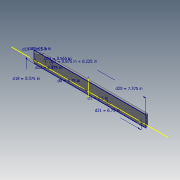
# Autodesk Inventor part: FLUGGER CAP SIDE FLUSH GUIDE
Saved by Autodesk Inventor 2020.3 (Build 243373000, 373)
## iProperties
RuleStatus: InUse
AfterDocSave0: file://Part Number Cleaner
Created: 2018-10-13
Material: Generic
Vendor: HHMI: JRC - ID&F
Document SubType Name: Modeling
Designer: arnoldj
Density: 1 g/cm^3
Appearance: Default
DESIGN DEPARTMENT: HHMI: JRC - ID&F
ALTERED ITEM PART NUMBER: N/A
ALTERED ITEM VENDOR: N/A
ALTERED ITEM DESCRIPTION: N/A
Author: arnoldj
Revision Number: 0
Autodesk Inventor part; units mm, degrees
ref_plane "YZ Plane" through (0, 0, 0) normal (1, 0, 0) x (0, 1, 0)
ref_plane "XZ Plane" through (0, 0, 0) normal (0, 1, 0) x (-1, 0, 0)
sketch "Sketch1" plane through (0, 0, 0) normal (0, 0, 1) x (1, 0, 0)
  line L0 (0, 35.433) -> (0, -17.018) projected
  line L1 (-250.825, 0) -> (260.35, 0) projected
  line L2 (187.325, -9.525) -> (-177.8, -9.525)
  line L3 (-177.8, -9.525) -> (-177.8, 27.94)
  line L4 (-177.8, 27.94) -> (187.325, 27.94)
  line L5 (187.325, 27.94) -> (187.325, -9.525)
  point P0 (0, 0)
  point P1 (-171.45, 0)
  point P2 (0, 0)
  point P3 (63.5, 0)
  point P4 (171.45, 0)
  point P5 (-139.7, 13.589)
  point P6 (-117.475, 13.589)
  dimension "d0" = 171.45
  dimension "d1" = 63.5
  dimension "d17" = 27.94
  dimension "d18" = 9.525
  dimension "d19" = 6.35
  dimension "d20" = 187.325
  dimension "d21" = 171.45
  dimension "d33" = 22.225
  dimension "d34" = 14.351
  dimension "d35" = 38.1
  constraints: 8 end point, 5 point on line, 2 parallel, 1 horizontal, 1 horizontal alignment, 1 perpendicular
  measures "d0" distance from line of L0 point (-171.45, 0)
  measures "d1" distance from line of L0 point (63.5, 0)
  measures "d17" distance between parallel lines of L1 L4
  measures "d18" distance between parallel lines of L2 L1
  measures "d19" distance from line of point (-171.45, 0) L3
  measures "d20" distance between parallel lines of L5 L0
  measures "d21" distance from line of L0 point (171.45, 0)
  measures "d33" distance of point (-139.7, 13.589) point (-117.475, 13.589)
  measures "d34" distance from line of L4 point (-117.475, 13.589)
  measures "d35" distance from line of L3 point (-139.7, 13.589)
extrude "Extrusion1" add sketch "Sketch1" against normal blind 6.35
sketch "Sketch2" plane through (0, 0, -6.35) normal (0, 0, -1) x (-1, 0, 0)
  point P0 (0, 0)
  point P1 (171.45, 0)
  point P2 (0, 0)
  point P3 (-63.5, 0)
  point P4 (-171.45, 0)
chamfer "Chamfer1" distance 25.4 angle 20 1 edges at (-177.8, 27.94, -3.175) measured on face at (-56.0917, 27.94, -2.1167)
fillet "Fillet1" radius 3.175 5 edges at (187.325, 27.94, -3.175) (187.325, -9.525, -3.175) (-177.8, -9.525, -3.175) (-177.8, 18.6952, -3.175) (-152.4, 27.94, -3.175)
hole "Hole2" [suppressed]
sketch "Sketch3" plane through (0, 0, 0) normal (0, 0, 1) x (1, 0, 0)
  line L0 (-171.45, -1.5875) -> (-171.45, 1.5875) construction
  line L1 (-168.91, -1.5875) -> (-168.91, 1.5875)
  line L2 (-173.99, 1.5875) -> (-173.99, -1.5875)
  arc A0 (-173.99, -1.5875) -> (-168.91, -1.5875) centre (-171.45, -1.5875) ccw
  arc A1 (-168.91, 1.5875) -> (-173.99, 1.5875) centre (-171.45, 1.5875) ccw
  line L3 (0, -1.5875) -> (0, 1.5875) construction
  line L4 (2.54, -1.5875) -> (2.54, 1.5875)
  line L5 (-2.54, 1.5875) -> (-2.54, -1.5875)
  arc A2 (-2.54, -1.5875) -> (2.54, -1.5875) centre (0, -1.5875) ccw
  arc A3 (2.54, 1.5875) -> (-2.54, 1.5875) centre (0, 1.5875) ccw
  line L6 (63.5, -1.5875) -> (63.5, 1.5875) construction
  line L7 (66.04, -1.5875) -> (66.04, 1.5875)
  line L8 (60.96, 1.5875) -> (60.96, -1.5875)
  arc A4 (60.96, -1.5875) -> (66.04, -1.5875) centre (63.5, -1.5875) ccw
  arc A5 (66.04, 1.5875) -> (60.96, 1.5875) centre (63.5, 1.5875) ccw
  line L9 (171.45, -1.5875) -> (171.45, 1.5875) construction
  line L10 (173.99, -1.5875) -> (173.99, 1.5875)
  line L11 (168.91, 1.5875) -> (168.91, -1.5875)
  arc A6 (168.91, -1.5875) -> (173.99, -1.5875) centre (171.45, -1.5875) ccw
  arc A7 (173.99, 1.5875) -> (168.91, 1.5875) centre (171.45, 1.5875) ccw
  point P0 (0, 0)
  point P1 (-171.45, 0)
  point P2 (0, 0)
  point P3 (63.5, 0)
  point P4 (171.45, 0)
  dimension "d29" = 2.54
  dimension "d30" = 3.175
  constraints: 32 end point, 16 point on circle, 16 tangent, 10 parallel, 8 centre point, 4 midpoint, 3 equal radius, 1 vertical
  measures "d29" radius of A1
  measures "d30" distance of L2.start L2.end
extrude "Extrusion2" cut sketch "Sketch3" against normal up to next
hole "Hole3" at (-139.7, 13.589, 0) at (-117.475, 13.589, 0) direction (0, 0, -1) diameter 3.1242 end through all
body "Solid1"
